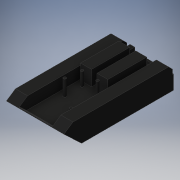
# Autodesk Inventor part: kocsi
Saved by Autodesk Inventor 2019 (Build 230136000, 136)
## iProperties
Created: 2019-02-10
Part Number: kocsi
Material: Generic
Document SubType Name: Modeling
Designer: izsoandras
Density: 1 g/cm^3
Appearance: Default
Author: izsoandras
Autodesk Inventor part; units mm, degrees
ref_plane "YZ Plane" through (0, 0, 0) normal (1, 0, 0) x (0, 1, 0)
ref_plane "XZ Plane" through (0, 0, 0) normal (0, 1, 0) x (-1, 0, 0)
ref_plane "XY Plane" through (0, 0, 0) normal (0, 0, 1) x (1, 0, 0)
sketch "Sketch1" plane through (0, 0, 0) normal (0, 1, 0) x (-1, 0, 0)
  line L0 (-45.0135, 84.3784) -> (49.9865, 84.3784)
  line L1 (49.9865, 84.3784) -> (49.9865, -94.6216)
  line L2 (49.9865, -94.6216) -> (-45.0135, -94.6216)
  line L3 (-45.0135, -94.6216) -> (-45.0135, 84.3784)
  point P0 (0, 0)
  dimension "d0" = 179
  dimension "d1" = 95
  constraints: 8 end point, 2 parallel, 1 horizontal, 1 perpendicular
  measures "d0" distance of L0.end L1.end
  measures "d1" distance of L1.end L2.end
extrude "test" add sketch "Sketch1" along normal blind 37.5
sketch "Sketch2" plane through (0, 37.5, 0) normal (0, 1, 0) x (1, 0, 0)
  line L0 (-29.9865, -83.3784) -> (25.0135, -83.3784)
  line L1 (25.0135, -83.3784) -> (25.0135, 93.6216)
  line L2 (25.0135, 93.6216) -> (-29.9865, 93.6216)
  line L3 (-29.9865, 93.6216) -> (-29.9865, -83.3784)
  line L4 (-49.9865, -84.3784) -> (45.0135, -84.3784) projected
  line L5 (-49.9865, 94.6216) -> (-49.9865, -84.3784) projected
  point P0 (0, 0)
  dimension "d4" = 55
  dimension "d5" = 177
  dimension "d6" = 1
  dimension "d7" = 20
  constraints: 8 end point, 2 parallel, 1 horizontal, 1 perpendicular
  measures "d4" distance of L0.start L0.end
  measures "d5" distance of L2.end L0.start
  measures "d6" distance between parallel lines of L4 L0
  measures "d7" distance between parallel lines of L5 L3
extrude "hasa" cut sketch "Sketch2" against normal blind 20
sketch "Sketch3" plane through (45.0135, 0, 84.3784) normal (1, 0, 0) x (0, 0, -1)
  line L0 (179, 37.5) -> (172.636, 37.5)
  line L1 (172.636, 37.5) -> (172.636, 37.5)
  line L2 (179, 31.136) -> (179, 31.136)
  line L3 (179, 31.136) -> (179, 37.5)
  line L4 (0, 37.5) -> (179, 37.5) projected
  line L5 (179, 0) -> (179, 37.5) projected
  line L6 (172.636, 37.5) -> (179, 31.136)
  point P0 (84.3784, 0)
  point P1 (172.636, 31.136)
  dimension "d10" = 6.364
  dimension "d11" = 6.364
  dimension "d12" = 0
  dimension "d13" = 0
  dimension "d14" = 6.364
  dimension "d15" = 45
  constraints: 10 end point, 2 parallel, 2 point on line, 1 horizontal, 1 perpendicular
  measures "d10" distance of point (172.636, 31.136) L2.end
  measures "d11" distance of L0.end point (172.636, 31.136)
  measures "d12" distance between parallel lines of L4 L0
  measures "d13" distance between parallel lines of L5 L3
  measures "d14" distance of L1.end point (172.636, 31.136)
  measures "d15" angle of L1 L6
extrude "hátsó levágás" cut sketch "Sketch3" against normal through all
sketch "Sketch4" plane through (45.0135, 0, -94.6216) normal (0, 0, -1) x (-1, 0, 0)
  line L0 (95, 0) -> (95, 37.5) projected
  line L1 (0, 0) -> (95, 0)
  line L2 (95, 0) -> (95, 23.136)
  line L3 (95, 23.136) -> (0, 23.136)
  line L4 (0, 23.136) -> (0, 0)
  line L5 (95, 31.136) -> (0, 31.136) projected
  point P0 (45.0135, 0)
  dimension "d18" = 8
  constraints: 8 end point, 2 parallel, 1 horizontal, 1 perpendicular, 1 point on line
  measures "d18" distance between parallel lines of L5 L3
extrude "hátsó kiszögellés" add sketch "Sketch4" along normal blind 2
sketch "Sketch6" plane through (45.0135, 31.136, -94.6216) normal (0, 0, -1) x (-1, 0, 0)
  line L0 (20, 1) -> (20, -13.636) projected
  line L1 (95, -8) -> (0, -8) projected
  line L2 (20, 1) -> (75, 1)
  line L3 (75, 1) -> (75, -8)
  line L4 (75, -8) -> (20, -8)
  line L5 (20, -8) -> (20, 1)
  line L6 (75, 1) -> (75, 6.364) projected
  line L7 (20, 1) -> (75, 1) projected
  point P0 (45.0135, -31.136)
  dimension "d21" = 0
  constraints: 8 end point, 2 parallel, 2 point on line, 1 collinear, 1 horizontal, 1 perpendicular
  measures "d21" distance between parallel lines of L7 L2
extrude "Extrusion5" cut sketch "Sketch6" against normal up to surface (1 mm away)
sketch "Sketch7" plane through (0, 17.5, 0) normal (0, 1, 0) x (1, 0, 0)
  line L0 (25.0135, 93.6216) -> (-29.9865, 93.6216) projected
  line L1 (-23.9865, 93.6216) -> (-15.9865, 93.6216)
  line L2 (-15.9865, 93.6216) -> (-15.9865, 79.6216)
  line L3 (-15.9865, 79.6216) -> (-23.9865, 79.6216)
  line L4 (-23.9865, 79.6216) -> (-23.9865, 93.6216)
  line L5 (-29.9865, -83.3784) -> (-29.9865, 88.2577) projected
  point P0 (0, 0)
  dimension "d24" = 14
  dimension "d25" = 8
  dimension "d26" = 6
  constraints: 8 end point, 2 parallel, 1 horizontal, 1 perpendicular, 1 point on line
  measures "d24" distance of L1.end L2.end
  measures "d25" distance of L2.end L3.end
  measures "d26" distance between parallel lines of L4 L5
extrude "táp csati" add sketch "Sketch7" along normal blind 15
sketch "Sketch8" plane through (45.0135, 0, 84.3784) normal (1, 0, 0) x (0, 0, -1)
  line L0 (0, 0) -> (0, 37.5) projected
  line L1 (0, 37.5) -> (15, 37.5)
  line L2 (15, 37.5) -> (15, 37.5)
  line L3 (0, 27.5) -> (0, 27.5)
  line L4 (0, 27.5) -> (0, 37.5)
  line L5 (15, 37.5) -> (0, 27.5)
  point P0 (84.3784, 0)
  point P1 (15, 27.5)
  dimension "d29" = 10
  dimension "d30" = 10
  dimension "d31" = 15
  dimension "d32" = 15
  constraints: 10 end point, 2 parallel, 2 point on line, 1 horizontal, 1 perpendicular
  measures "d29" distance of L1.end point (15, 27.5)
  measures "d30" distance of L2.end point (15, 27.5)
  measures "d31" distance of L3.start point (15, 27.5)
  measures "d32" distance of L0.end L1.end
extrude "első levágás" cut sketch "Sketch8" against normal through all
sketch "Sketch9" plane through (0, 17.5, 0) normal (0, 1, 0) x (1, 0, 0)
  line L0 (-27.9865, 79.1216) -> (-9.9865, 79.1216)
  line L1 (-9.9865, 79.1216) -> (-9.9865, 16.1216)
  line L2 (-9.9865, 16.1216) -> (-27.9865, 16.1216)
  line L3 (-27.9865, 16.1216) -> (-27.9865, 79.1216)
  line L4 (-29.9865, -69.3784) -> (-29.9865, 88.2577) projected
  line L5 (25.0135, 93.6216) -> (-15.9865, 93.6216) projected
  line L6 (25.0135, 88.2577) -> (25.0135, -69.3784) projected
  point P0 (0, 0)
  dimension "d35" = 63
  dimension "d36" = 18
  dimension "d37" = 2
  dimension "d38" = 14.5
  constraints: 8 end point, 2 parallel, 1 horizontal, 1 perpendicular
  measures "d35" distance of L0.end L1.end
  measures "d36" distance of L1.end L2.end
  measures "d37" distance between parallel lines of L4 L3
  measures "d38" distance between parallel lines of L5 L0
extrude "motor jobb" add sketch "Sketch9" along normal blind 25
sketch "Sketch10" plane through (0, 17.5, 0) normal (0, 1, 0) x (1, 0, 0)
  line L0 (0.0135, 79.1216) -> (18.0135, 79.1216)
  line L1 (18.0135, 79.1216) -> (18.0135, 15.1216)
  line L2 (18.0135, 15.1216) -> (0.0135, 15.1216)
  line L3 (0.0135, 15.1216) -> (0.0135, 79.1216)
  line L4 (25.0135, 88.2577) -> (25.0135, -69.3784) projected
  line L5 (25.0135, 93.6216) -> (-15.9865, 93.6216) projected
  point P0 (0, 0)
  dimension "d45" = 7
  dimension "d46" = 18
  dimension "d47" = 64
  dimension "d48" = 14.5
  constraints: 8 end point, 2 parallel, 1 horizontal, 1 perpendicular
  measures "d45" distance between parallel lines of L4 L1
  measures "d46" distance between parallel lines of L3 L1
  measures "d47" distance of L2.end L0.start
  measures "d48" distance between parallel lines of L5 L0
extrude "motor bal" add sketch "Sketch10" along normal blind 25
sketch "Sketch11" plane through (45.0135, 0, -96.6216) normal (1, 0, 0) x (0, 0, -1)
  line L0 (-181, 0) -> (-181, 27.5) projected
  line L1 (-181, 27.5) -> (-151.8278, 0)
  line L2 (0, 0) -> (-181, 0) projected
  line L3 (-166, 37.5) -> (-181, 27.5) projected
  point P0 (-96.6216, 0)
  dimension "d51" = 77
  constraints: 2 end point, 1 point on line
  measures "d51" angle of L3 L1
extrude "eleje alső levágás" cut sketch "Sketch11" against normal through all
sketch "Sketch12" plane through (-29.9865, 23.136, -94.6216) normal (1, 0, 0) x (0, 0, -1)
  line L0 (-168.3919, -5.636) -> (-1, -5.636) projected
  line L1 (-178, 3.4213) -> (-168.3919, -5.636) projected
  line L2 (-168.3919, -5.636) -> (-178, 3.4213)
  line L3 (-178, 3.4213) -> (-176.7937, 4.7009)
  line L4 (-176.7937, 4.7009) -> (-165.8282, -5.636)
  line L5 (-167.1856, -4.3564) -> (-168.3919, -5.636)
  line L6 (-164, 14.364) -> (-178, 5.0306) projected
  line L7 (-176.7937, 4.7009) -> (-178, 5.0306)
  line L8 (-178, 5.0306) -> (-178, 3.4213)
  line L9 (-168.3919, -5.636) -> (-165.8282, -5.636)
  point P0 (-94.6216, -23.136)
  constraints: 14 end point, 2 parallel, 2 perpendicular, 2 point on line, 1 collinear, 1 vertical
extrude "eleje korrekció" add sketch "Sketch12" along normal up to next
sketch "Sketch13" plane through (0, 17.5, 0) normal (0, 1, 0) x (1, 0, 0)
  circle A0 centre (-18.7965, -19.1834) radius 2.3
  line L0 (-29.9865, -69.3784) -> (-29.9865, 88.2577) projected
  line L1 (-29.9865, -83.3784) -> (25.0135, -83.3784) projected
  point P0 (0, 0)
  dimension "d56" = 4.6
  dimension "d57" = 11.19
  dimension "d58" = 64.195
  constraints: 1 centre point
  measures "d56" diameter of A0
  measures "d57" distance from line of L0 A0.centre
  measures "d58" distance from line of L1 A0.centre
extrude "oszlop1" add sketch "Sketch13" along normal blind 26.01
sketch "Sketch14" plane through (0, 17.5, 0) normal (0, 1, 0) x (1, 0, 0)
  circle A0 centre (-18.9886, 9.4943) radius 2.3
  point P0 (0, 0)
  dimension "d61" = 4.6
  constraints: 1 centre point
  measures "d61" diameter of A0
extrude "oszlop2" add sketch "Sketch14" along normal blind 22.3
sketch "Sketch15" plane through (0, 17.5, 0) normal (0, 1, 0) x (1, 0, 0)
  circle A0 centre (7.9502, 8.1031) radius 2.205
  point P0 (0, 0)
  dimension "d64" = 4.41
  constraints: 1 centre point
  measures "d64" diameter of A0
extrude "oszlop3" add sketch "Sketch15" along normal blind 22.2
sketch "Sketch16" plane through (0, 17.5, 0) normal (0, 1, 0) x (1, 0, 0)
  circle A0 centre (13.5812, -41.274) radius 2.35
  point P0 (0, 0)
  dimension "d67" = 4.7
  constraints: 1 centre point
  measures "d67" diameter of A0
extrude "oszlop4" add sketch "Sketch16" along normal blind 10.12
equation "\"d11\" = d10"
equation "\"d14\" = d10"
body "Solid1"
